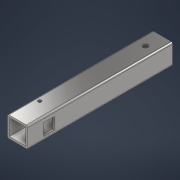
# Autodesk Inventor part: member_transverse_inner
Saved by Autodesk Inventor 2021 (Build 250183000, 183)
## iProperties
Created: 2021-06-01
Part Number: member_transverse_inner
Material: Steel, Galvanized
Document SubType Name: Modeling
Designer: Watchdog
Density: 7.85 g/cm^3
Appearance: Galvanized
Mass: 278.238 g
Surface Area: 293.624 cm^2
Volume: 35.4444 cm^3
Author: Watchdog
Autodesk Inventor part; units mm, degrees
ref_plane "YZ Plane" through (0, 0, 0) normal (1, 0, 0) x (0, 1, 0)
ref_plane "XZ Plane" through (0, 0, 0) normal (0, 1, 0) x (-1, 0, 0)
ref_plane "XY Plane" through (0, 0, 0) normal (0, 0, 1) x (1, 0, 0)
sketch "Sketch1" plane through (0, 0, 0) normal (0, 0, 1) x (1, 0, 0)
  line L0 (-12.25, 12.25) -> (12.25, 12.25)
  line L1 (12.25, 12.25) -> (12.25, -12.25)
  line L2 (12.25, -12.25) -> (-12.25, -12.25)
  line L3 (-12.25, -12.25) -> (-12.25, 12.25)
  line L4 (9.75, 9.75) -> (-9.75, 9.75)
  line L5 (-9.75, 9.75) -> (-9.75, -9.75)
  line L6 (-9.75, -9.75) -> (9.75, -9.75)
  line L7 (9.75, -9.75) -> (9.75, 9.75)
  point P0 (0, 0)
  dimension "d0" = 24.5
  dimension "d1" = 24.5
  dimension "d2" = 12.25
  dimension "d3" = 12.25
  dimension "d4" = 2.5
  constraints: 16 end point, 4 parallel, 2 perpendicular, 1 horizontal, 3 other
  measures "d0" distance of L0.start L0.end
  measures "d1" distance of L2.end L0.start
  measures "d2" distance from line of point (0, 0) L0
  measures "d3" distance from line of point (0, 0) L3
  measures "d4" distance between parallel lines of L0 L4
extrude "Extrusion1" add sketch "Sketch1" along normal blind 1000
fillet "Fillet1" radius 2 4 edges at (12.25, 12.25, 500) (-12.25, 12.25, 500) (-12.25, -12.25, 500) (12.25, -12.25, 500)
ref_plane "endPlane" through (0, 0, 172.25) normal (0, 0, -1) x (-1, 0, 0)
split "Split1" plane through (0, 0, 172.25) removes the side toward (0, 0, 1)
ref_plane "midPlane" through (-10.25, -12.25, 86.125) normal (0, 0, 1) x (1, 0, 0)
sketch "Sketch2" plane through (-10.25, 12.25, 0) normal (0, 1, 0) x (1, 0, 0)
  line L0 (10.25, -20) -> (10.25, -20) construction
  line L1 (13.25, -20) -> (13.25, -20)
  line L2 (7.25, -20) -> (7.25, -20)
  arc A0 (7.25, -20) -> (13.25, -20) centre (10.25, -20) ccw
  arc A1 (13.25, -20) -> (7.25, -20) centre (10.25, -20) ccw
  point P0 (10.25, 0)
  point P1 (10.25, -40)
  dimension "d46" = 6
  dimension "d47" = 0
  dimension "d48" = 20
  dimension "d49" = 0
  constraints: 8 end point, 4 point on circle, 4 tangent, 2 centre point, 1 parallel, 1 point on line, 1 vertical
  measures "d46" diameter of A1
  measures "d47" horizontal distance of point (10.25, 0) L0.end
  measures "d48" distance of L0.end point (10.25, 0)
  measures "d49" distance of L0.end L0.start
sketch "Sketch3" plane through (12.25, -10.25, 0) normal (1, 0, 0) x (0, 0, -1)
  line L0 (-153.75, 16.4128) -> (-140.75, 16.4128)
  line L1 (-140.75, 16.4128) -> (-140.75, 2.4128)
  line L2 (-140.75, 2.4128) -> (-153.75, 2.4128)
  line L3 (-153.75, 2.4128) -> (-153.75, 16.4128)
  line L4 (-172.25, 20.5) -> (-172.25, 0) projected
  point P0 (0, 10.25)
  dimension "d28" = 14
  dimension "d29" = 18.5
  dimension "d30" = 13
  constraints: 8 end point, 2 parallel, 1 horizontal, 1 perpendicular
  measures "d28" distance between parallel lines of L2 L0
  measures "d29" distance between parallel lines of L4 L3
  measures "d30" distance between parallel lines of L3 L1
extrude "Extrusion2" cut sketch "Sketch3" against normal up to surface (2.5 mm away)
sketch "Sketch4" plane through (-10.25, 12.25, 0) normal (0, 1, 0) x (1, 0, 0)
  line L0 (-2, 0) -> (-2, -1000) projected
  line L1 (0, -172.25) -> (20.5, -172.25) projected
  point P0 (10.25, 0)
  point P1 (-2, -172.25)
  point P2 (4, -139.75)
  point P3 (22.5, -140.75)
  dimension "d36" = 6
  dimension "d45" = 1
  measures "d36" distance from line of L0 point (4, -139.75)
  measures "d45" vertical distance of point (22.5, -140.75) point (4, -139.75)
hole "Hole2" at (-6.25, 12.25, 139.75) direction (0, -1, 0) diameter 4 end through all
ref_plane "Work Plane3" through (12.25, -7.8372, 147.25) normal (0, 0, 1) x (1, 0, 0)
extrude "Extrusion3" cut sketch "Sketch2" against normal through all
equation "\"d0\" = -2 * a + sm_varx_squareBarDimension - tol"
equation "\"d1\" = d0"
equation "\"d2\" = 0.5 * d1"
equation "\"d3\" = 0.5 * d0"
equation "\"d4\" = sm_varx_squareBarThickness"
equation "\"d8\" = -sm_varx_z - 0.5 * d0"
equation "\"sm_varx_squareBarThickness\" = 2.5"
equation "\"sm_varx_pinPlate_holeDiameter\" = 5"
equation "\"sm_varx_member_tolerance\" = 0.5"
equation "\"a\" = sm_varx_squareBarThickness"
equation "\"tol\" = sm_varx_member_tolerance"
equation "\"hoop_angle_z\" = 45deg"
equation "\"hoop_bearing_length\" = 5deg"
equation "\"hoop_cable_diam\" = 5"
equation "\"hoop_cable_pulley_diam\" = 22"
equation "\"hoop_thickness_large\" = 4"
equation "\"hoop_thickness_medium\" = 3.2"
equation "\"hoop_thickness_small\" = 2"
equation "\"hoop_width_large\" = 51"
equation "\"hoop_width_medium\" = 33.7"
equation "\"hoop_width_small\" = 25.4"
equation "\"rack_tooth_addendum\" = 5"
equation "\"rack_tooth_dedendum\" = 5"
equation "\"rack_tooth_thickness\" = 5"
equation "\"secure_arm_angle\" = 35deg"
equation "\"secure_arm_radii\" = 9"
equation "\"support_baseClamp_platformLengthBuffer\" = 35"
equation "\"support_baseClamp_platformThickness\" = 15"
equation "\"support_baseClamp_platformWidthBuffer\" = 0"
equation "\"support_baseClamp_sleeveHoleDiameter\" = 12"
equation "\"support_baseClamp_sleeveSweepTerminationAngle\" = 55deg"
equation "\"support_baseClamp_thickness\" = 8"
equation "\"support_frame_endHoleBuffer\" = 25"
equation "\"support_frame_squareBarFillet\" = 2"
equation "\"support_frame_squareBarThickness\" = 5"
equation "\"hoop_tabs_thickness\" = 6"
equation "\"hoop_tabs_hole\" = 12"
equation "\"wheelchair_deployed_width\" = 635"
equation "\"wheelchair_deployed_length\" = 1067"
equation "\"wheelchair_deployed_height\" = 914"
equation "\"sm_varx_pinPlate_thickness\" = 5"
equation "\"hoop_bushing12_radialInterference\" = 0"
equation "\"hoop_bushing23_radialInterference\" = 0"
equation "\"hoop_bushing23_od\" = -2 * hoop_thickness_medium + hoop_width_medium + hoop_bushing23_radialInterference"
equation "\"sm_varx_squareBarDimension\" = 30"
equation "\"sm_varx_z\" = 160"
body "Solid1"
